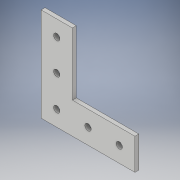
# Autodesk Inventor part: L-Guesset
Saved by Autodesk Inventor 2018 (Build 220112000, 112)
## iProperties
Created: 2020-01-26
Part Number: L-Guesset
Material: Generic
Document SubType Name: Modeling
Designer: maste
Density: 1 g/cm^3
Appearance: Default
Author: maste
Autodesk Inventor part; units mm, degrees
ref_plane "YZ Plane" through (0, 0, 0) normal (1, 0, 0) x (0, 1, 0)
ref_plane "XZ Plane" through (0, 0, 0) normal (0, 1, 0) x (-1, 0, 0)
ref_plane "XY Plane" through (0, 0, 0) normal (0, 0, 1) x (1, 0, 0)
sketch "Sketch1" plane through (0, 0, 0) normal (0, 0, 1) x (1, 0, 0)
  line L0 (0, 0) -> (25.4, 0)
  line L1 (25.4, 25.4) -> (25.4, 76.2)
  line L2 (25.4, 76.2) -> (0, 76.2)
  line L3 (0, 76.2) -> (0, 0)
  line L4 (0, 0) -> (76.2, 0)
  line L5 (76.2, 0) -> (76.2, 25.4)
  line L6 (76.2, 25.4) -> (25.4, 25.4)
  line L7 (0, 25.4) -> (0, 0)
  line L8 (12.7, 76.2) -> (12.7, 63.5) construction
  line L9 (12.7, 63.5) -> (12.7, 38.1) construction
  line L10 (12.7, 38.1) -> (12.7, 12.7) construction
  line L11 (12.7, 12.7) -> (38.1, 12.7) construction
  line L12 (38.1, 12.7) -> (63.5, 12.7) construction
  circle A0 centre (12.7, 63.5) radius 2.5797
  circle A1 centre (12.7, 38.1) radius 2.5797
  circle A2 centre (12.7, 12.7) radius 2.5797
  circle A3 centre (38.1, 12.7) radius 2.5797
  circle A4 centre (63.5, 12.7) radius 2.5797
  dimension "d0" = 25.4
  dimension "d1" = 76.2
  dimension "d2" = 76.2
  dimension "d3" = 25.4
  dimension "d4" = 12.7
  dimension "d5" = 25.4
  dimension "d6" = 25.4
  dimension "d7" = 25.4
  dimension "d8" = 25.4
  dimension "d9" = 5.1594
  constraints: 26 end point, 5 centre point, 5 coincident, 4 parallel, 3 perpendicular, 3 point on line, 2 horizontal, 1 midpoint, 1 vertical
  measures "d0" distance of L2.end L1.end
  measures "d1" distance of L1.end L0.end
  measures "d2" distance of L7.start L5.end
  measures "d3" distance of L5.end L4.end
  measures "d4" distance of L8.start L8.end
  measures "d5" distance of L8.end L9.end
  measures "d6" distance of L9.end L10.end
  measures "d7" distance of L10.end L11.end
  measures "d8" distance of L11.end L12.end
  measures "d9" diameter of A0
extrude "Extrusion1" add sketch "Sketch1" along normal blind 3.175
body "Solid1"
